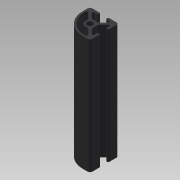
# Autodesk Inventor part: 25-2527-BLACK-FB
Saved by Autodesk Inventor 2013 (Build 170138000, 138)
## iProperties
Company: 80/20 Inc.
Created: 2014-04-23
Part Number: 25-2527-BLACK-FB
Material: Generic
Document SubType Name: Modeling
Designer: Ross Bowman
Density: 1 g/cm^3
Engineer: Ross Bowman
Catalog Web Link: 8020.net
Vendor: 80/20 Inc.
Material: 6105-T5 Aluminum
Author: Ross Bowman
Keywords: 80/20 , 8020 , T-Slot , Extrusion
Autodesk Inventor part; units mm, degrees
ref_plane "YZ Plane" through (0, 0, 0) normal (1, 0, 0) x (0, 1, 0)
ref_plane "XZ Plane" through (0, 0, 0) normal (0, 1, 0) x (-1, 0, 0)
ref_plane "XY Plane" through (0, 0, 0) normal (0, 0, 1) x (1, 0, 0)
sketch "Sketch1" plane through (0, 0, 0) normal (0, 0, 1) x (1, 0, 0)
  arc A0 (-10.9617, 7.0429) -> (7.0429, -10.9617) centre (6.25, 6.25) ccw
  arc A1 (-9.228, 7.7147) -> (-10.9617, 7.0429) centre (-9.9466, 6.9961) ccw
  line L0 (-4.9841, 3.4709) -> (-9.228, 7.7147)
  arc A2 (-4.054, 1.2253) -> (-4.9841, 3.4709) centre (-7.2298, 1.2253) ccw
  line L1 (-4.054, 0) -> (-4.054, 1.2253)
  arc A3 (-4.054, 0) -> (0, -4.054) centre (0, 0) ccw
  line L2 (1.2253, -4.054) -> (0, -4.054)
  arc A4 (3.4709, -4.9841) -> (1.2253, -4.054) centre (1.2253, -7.2298) ccw
  line L3 (7.7147, -9.228) -> (3.4709, -4.9841)
  arc A5 (7.0429, -10.9617) -> (7.7147, -9.228) centre (6.9961, -9.9466) ccw
  circle A6 centre (0, 0) radius 2.5
  arc A7 (5.2692, 3.756) -> (4.4, 1.6576) centre (7.3675, 1.6576) ccw
  line L4 (5.2692, 3.756) -> (8.6136, 7.1004)
  arc A8 (10.36, 6.377) -> (8.6136, 7.1004) centre (9.337, 6.377) ccw
  line L5 (10.36, 6.377) -> (10.36, 4.32)
  arc A9 (10.36, 4.32) -> (12.5, 4.32) centre (11.43, 4.32) ccw
  line L6 (12.5, 4.32) -> (12.5, 10.5209)
  arc A10 (12.5, 10.5209) -> (10.5209, 12.5) centre (10.5209, 10.5209) ccw
  line L7 (10.5209, 12.5) -> (4.32, 12.5)
  arc A11 (4.32, 12.5) -> (4.32, 10.36) centre (4.32, 11.43) ccw
  line L8 (4.32, 10.36) -> (6.377, 10.36)
  arc A12 (7.1004, 8.6136) -> (6.377, 10.36) centre (6.377, 9.337) ccw
  line L9 (7.1004, 8.6136) -> (3.6484, 5.1617)
  arc A13 (1.6576, 4.39) -> (3.6484, 5.1617) centre (1.6576, 7.344) ccw
  line L10 (1.6576, 4.39) -> (-1.6576, 4.39)
  arc A14 (-3.6484, 5.1617) -> (-1.6576, 4.39) centre (-1.6576, 7.344) ccw
  line L11 (-3.6484, 5.1617) -> (-7.1004, 8.6136)
  arc A15 (-6.377, 10.36) -> (-7.1004, 8.6136) centre (-6.377, 9.337) ccw
  line L12 (-6.377, 10.36) -> (-4.32, 10.36)
  arc A16 (-4.32, 10.36) -> (-4.32, 12.5) centre (-4.32, 11.43) ccw
  line L13 (-4.32, 12.5) -> (-10.5209, 12.5)
  arc A17 (-10.5209, 12.5) -> (-12.5, 10.5209) centre (-10.5209, 10.5209) ccw
  line L14 (-12.5, 10.5209) -> (-12.5, 6.25)
  arc A18 (-12.5, 6.25) -> (6.25, -12.5) centre (6.25, 6.25) ccw
  line L15 (6.25, -12.5) -> (10.5209, -12.5)
  arc A19 (10.5209, -12.5) -> (12.5, -10.5209) centre (10.5209, -10.5209) ccw
  line L16 (12.5, -10.5209) -> (12.5, -4.32)
  arc A20 (12.5, -4.32) -> (10.36, -4.32) centre (11.43, -4.32) ccw
  line L17 (10.36, -4.32) -> (10.36, -6.377)
  arc A21 (8.6136, -7.1004) -> (10.36, -6.377) centre (9.337, -6.377) ccw
  line L18 (8.6136, -7.1004) -> (5.2692, -3.756)
  arc A22 (4.4, -1.6576) -> (5.2692, -3.756) centre (7.3675, -1.6576) ccw
  line L19 (4.4, -1.6576) -> (4.4, 1.6576)
  constraints: 44 point on circle, 40 end point, 23 centre point
extrude "Extrusion1" add sketch "Sketch1" against normal blind 100
body "Solid1"
